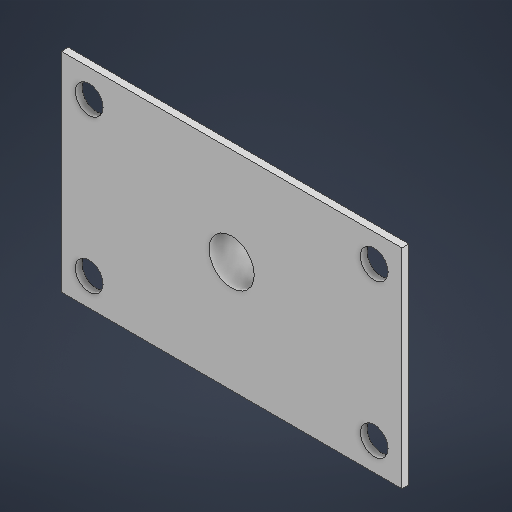
# Autodesk Inventor part: Potihalter
Saved by Autodesk Inventor 2026.2 (Build 302298000, 298)
## iProperties
Created: 2025-12-29
Part Number: Potihalter
Material: Generisch
Document SubType Name: Modeling
Designer: danie
Density: 1 g/cm^3
Appearance: Vorgabe
Author: danie
Autodesk Inventor part; units mm, degrees
ref_plane "YZ Plane" through (0, 0, 0) normal (1, 0, 0) x (0, 1, 0)
ref_plane "XZ Plane" through (0, 0, 0) normal (0, 1, 0) x (-1, 0, 0)
ref_plane "XY Plane" through (0, 0, 0) normal (0, 0, 1) x (1, 0, 0)
sketch "Skizze1" plane through (0, 0, 0) normal (0, 0, 1) x (1, 0, 0)
  line L0 (0, 30) -> (49, 30)
  line L1 (49, 30) -> (49, 0)
  line L2 (49, 0) -> (0, 0)
  line L3 (0, 0) -> (0, 30)
  line L4 (-9.8, 0) -> (58.8, 0) projected
  line L5 (0, -6) -> (0, 36) projected
  point P0 (0, 0)
  dimension "d0" = 49
  dimension "d1" = 30
  constraints: 8 end point, 2 collinear, 2 parallel, 1 horizontal, 1 perpendicular
  measures "d0" distance between parallel lines of L1 L3
  measures "d1" distance between parallel lines of L0 L2
extrude "Extrusion1" add sketch "Skizze1" along normal blind 1
sketch "Skizze2" plane through (0, 0, 0) normal (0, 0, -1) x (-1, 0, 0)
  circle A0 centre (-24.5, 16) radius 3.25
  line L0 (-49, 30) -> (0, 30) projected
  line L1 (0, 0) -> (-49, 0) projected
  circle A1 centre (-24.5, 16) radius 5.25
  line L2 (-41, 30) -> (-8, 30)
  line L3 (-8, 30) -> (-8, 2)
  line L4 (-8, 2) -> (-41, 2)
  line L5 (-41, 2) -> (-41, 30)
  line L6 (-49, 0) -> (-49, 30) projected
  line L7 (0, 30) -> (0, 0) projected
  line L8 (-24.5, 30) -> (-24.5, 2)
  dimension "d4" = 6.5
  dimension "d5" = 10.5
  dimension "d8" = 2
  dimension "d9" = 8
  dimension "d10" = 8
  dimension "d11" = 14
  constraints: 10 end point, 3 midpoint, 2 centre point, 2 parallel, 1 collinear, 1 concentric, 1 horizontal, 1 perpendicular
  measures "d4" diameter of A0
  measures "d5" diameter of A1
  measures "d8" distance between parallel lines of L1 L4
  measures "d9" distance between parallel lines of L6 L5
  measures "d10" distance between parallel lines of L7 L3
  measures "d11" distance from line of L4 A0.centre
extrude "Extrusion2" add sketch "Skizze2" along normal blind 6 contours A0 L8 A1 | A0 L8 A1
sketch "Skizze6" plane through (24.5, 16, 0) normal (0, 0, -1) x (-1, 0, 0)
  circle A0 centre (0, 0) radius 3.25
  circle A1 centre (0, 0) radius 3.25 projected
  point P0 (24.5, -16)
  constraints: 2 concentric, 1 centre point
extrude "Extrusion3" cut sketch "Skizze6" against normal through all
sketch "Skizze7" plane through (0, 0, 1) normal (0, 0, 1) x (1, 0, 0)
  line L0 (0, 30) -> (0, 0) projected
  line L1 (49, 30) -> (0, 30) projected
  point P0 (4, 26)
  point P1 (45, 26)
  point P2 (4, 4)
  point P3 (45, 4)
  dimension "d15" = 4
  dimension "d16" = 4
  dimension "d19" = 41
  dimension "d22" = 22
  constraints: 1 horizontal, 1 vertical, 3 other
  measures "d15" distance from line of L0 point (4, 26)
  measures "d16" distance from line of L1 point (4, 26)
  measures "d19" distance of point (4, 26) point (45, 26)
  measures "d22" distance of point (4, 26) point (4, 4)
hole "Bohrung1" at (4, 26, 1) at (45, 26, 1) at (4, 4, 1) at (45, 4, 1) direction (0, 0, -1) diameter 4 end through all
